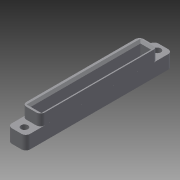
# Autodesk Inventor part: Part1
Saved by Autodesk Inventor 2015 (Build 190159000, 159)
## iProperties
Created: 2015-06-15
Part Number: Part1
Material: Generic
Document SubType Name: Modeling
Designer: smkilani
Density: 1 g/cm^3
Appearance: Default
Author: smkilani
Autodesk Inventor part; units mm, degrees
ref_plane "YZ Plane" through (0, 0, 0) normal (1, 0, 0) x (0, 1, 0)
ref_plane "XZ Plane" through (0, 0, 0) normal (0, 1, 0) x (-1, 0, 0)
ref_plane "XY Plane" through (0, 0, 0) normal (0, 0, 1) x (1, 0, 0)
sketch "Sketch1" plane through (0, 0, 0) normal (0, 1, 0) x (-1, 0, 0)
  line L0 (2.5675, -34.392) -> (-2.0625, -34.392)
  line L1 (-4.0625, -32.392) -> (-4.0625, 32.768)
  line L2 (-2.0625, 34.768) -> (2.5675, 34.768)
  line L3 (4.5675, 32.768) -> (4.5675, -32.392)
  arc A0 (4.5675, 32.768) -> (2.5675, 34.768) centre (2.5675, 32.768) ccw
  arc A1 (-2.0625, 34.768) -> (-4.0625, 32.768) centre (-2.0625, 32.768) ccw
  arc A2 (-4.0625, -32.392) -> (-2.0625, -34.392) centre (-2.0625, -32.392) ccw
  arc A3 (2.5675, -34.392) -> (4.5675, -32.392) centre (2.5675, -32.392) ccw
  point P0 (0, 0)
  point P1 (-4.0625, 34.768)
  point P2 (-4.0625, -34.392)
  point P3 (4.5675, 34.768)
  dimension "d0" = 8.63
  dimension "d1" = 69.16
  dimension "d2" = 2
  constraints: 8 end point, 8 point on circle, 8 tangent, 6 point on line, 4 centre point, 3 equal radius, 2 parallel, 1 horizontal, 1 perpendicular
  measures "d0" distance of point (-4.063, 34.768) point (4.567, 34.768)
  measures "d1" distance of point (-4.063, -34.392) point (-4.063, 34.768)
  measures "d2" radius of A0
extrude "Extrusion1" add sketch "Sketch1" along normal blind 6.35
sketch "Sketch2" plane through (0, 6.35, 0) normal (0, 1, 0) x (1, 0, 0)
  circle A0 centre (0, -31.355) radius 1.625
  circle A1 centre (0, 31.355) radius 1.625
  point P0 (0, 0)
  dimension "d5" = 3.25
  dimension "d6" = 3.25
  dimension "d7" = 31.355
  dimension "d8" = 31.355
  constraints: 2 centre point
  measures "d5" diameter of A0
  measures "d6" diameter of A1
  measures "d7" distance of point (0, 0) A0.centre
  measures "d8" distance of point (0, 0) A1.centre
extrude "Extrusion2" cut sketch "Sketch2" against normal blind 6.35
sketch "Sketch3" plane through (0, 6.35, 0) normal (0, 1, 0) x (1, 0, 0)
  line L0 (-2.569, -27.838) -> (2.061, -27.838)
  line L1 (4.061, -25.838) -> (4.061, 25.462)
  line L2 (2.061, 27.462) -> (-2.569, 27.462)
  line L3 (-4.569, 25.462) -> (-4.569, -25.838)
  line L4 (-2.5675, -34.768) -> (2.0625, -34.768) projected
  arc A0 (-4.569, -25.838) -> (-2.569, -27.838) centre (-2.569, -25.838) ccw
  arc A1 (2.061, -27.838) -> (4.061, -25.838) centre (2.061, -25.838) ccw
  arc A2 (4.061, 25.462) -> (2.061, 27.462) centre (2.061, 25.462) ccw
  arc A3 (-2.569, 27.462) -> (-4.569, 25.462) centre (-2.569, 25.462) ccw
  point P0 (0, 0)
  point P1 (4.061, 27.462)
  point P2 (4.061, -27.838)
  point P3 (-4.569, 27.462)
  dimension "d11" = 8.63
  dimension "d12" = 55.3
  dimension "d13" = 6.93
  dimension "d14" = 2
  constraints: 8 end point, 8 point on circle, 8 tangent, 6 point on line, 4 centre point, 3 equal radius, 2 parallel, 1 horizontal, 1 perpendicular
  measures "d11" distance of point (-4.569, 27.462) point (4.061, 27.462)
  measures "d12" distance of point (4.061, 27.462) point (4.061, -27.838)
  measures "d13" distance between parallel lines of L4 L0
  measures "d14" radius of A0
extrude "Extrusion3" add sketch "Sketch3" along normal blind 5.28
sketch "Sketch4" plane through (0, 11.63, 0) normal (0, 1, 0) x (1, 0, 0)
  line L0 (2.5, 25.855) -> (-2.5, 25.855)
  line L1 (-2.5, 25.855) -> (-2.5, -25.855)
  line L2 (-2.5, -25.855) -> (2.5, -25.855)
  line L3 (2.5, -25.855) -> (2.5, 25.855)
  line L4 (2.5, 25.855) -> (-2.5, -25.855) construction
  line L5 (-2.5, 25.855) -> (2.5, -25.855) construction
  point P0 (0, 0)
  dimension "d17" = 5
  dimension "d18" = 51.71
  constraints: 12 end point, 2 midpoint, 2 parallel, 1 horizontal, 1 perpendicular
  measures "d17" distance of L2.end L1.end
  measures "d18" distance of L1.end L0.end
extrude "Extrusion4" cut sketch "Sketch4" against normal blind 11.63
chamfer "Chamfer1" distance 1 angle 45 4 edges at (-2.5, 11.63, 0) (0, 11.63, 25.855) (2.5, 11.63, 0) (0, 11.63, -25.855)
sketch "Sketch5" plane through (0, 0, 0) normal (0, -1, 0) x (1, 0, 0)
  point P0 (0, 0)
body "Solid1"
